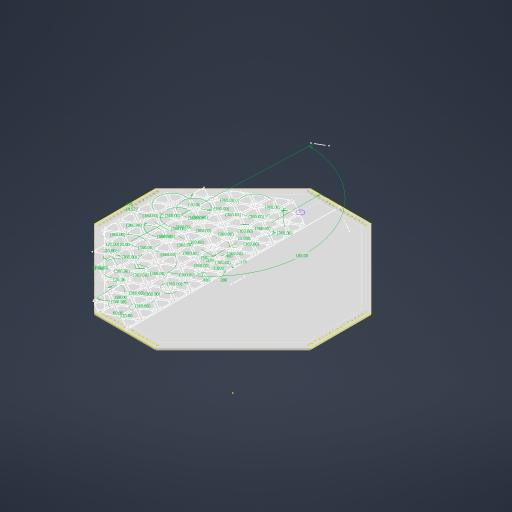
# Autodesk Inventor part: Belly Pan
Saved by Autodesk Inventor 2024.3 (Build 283343000, 343)
## iProperties
Created: 2024-11-27
Part Number: Belly Pan
Material: Generic
Document SubType Name: Modeling
Designer: kaito
Density: 1 g/cm^3
Appearance: Default
Author: kaito
Autodesk Inventor part; units mm, degrees
(part 1 of 3)
ref_plane "YZ Plane" through (0, 0, 0) normal (1, 0, 0) x (0, 1, 0)
ref_plane "XZ Plane" through (0, 0, 0) normal (0, 1, 0) x (-1, 0, 0)
ref_plane "XY Plane" through (0, 0, 0) normal (0, 0, 1) x (1, 0, 0)
sketch "Sketch1" plane through (0, 0, 0) normal (0, 1, 0) x (-1, 0, 0)
  line L0 (0, 0) -> (762, 0) construction
  line L1 (762, 0) -> (762, -762)
  line L2 (762, -762) -> (0, -762)
  line L3 (762, -273.05) -> (736.6, -273.05) construction
  line L4 (736.6, -273.05) -> (736.6, -488.95) construction
  line L5 (736.6, -488.95) -> (762, -488.95) construction
  line L6 (762, -488.95) -> (762, -273.05) construction
  line L7 (488.95, 0) -> (273.05, 0)
  line L8 (273.05, 0) -> (273.05, -25.4) construction
  line L9 (273.05, -25.4) -> (488.95, -25.4) construction
  line L10 (488.95, -25.4) -> (488.95, 0) construction
  line L11 (488.95, -762) -> (273.05, -762) construction
  line L12 (273.05, -762) -> (273.05, -736.6) construction
  line L13 (273.05, -736.6) -> (488.95, -736.6) construction
  line L14 (488.95, -736.6) -> (488.95, -762) construction
  line L15 (0, 0) -> (0, -762)
  line L16 (0, -273.05) -> (25.4, -273.05) construction
  line L17 (25.4, -273.05) -> (25.4, -488.95) construction
  line L18 (25.4, -488.95) -> (0, -488.95) construction
  line L19 (0, -488.95) -> (0, -273.05) construction
  line L20 (273.05, 0) -> (0, -273.05)
  line L21 (488.95, 0) -> (762, -273.05)
  line L22 (762, -488.95) -> (488.95, -762)
  line L23 (0, -488.95) -> (273.05, -762)
  circle A0 centre (482.6, -12.7) radius 2.4892
  circle A1 centre (469.9, -12.7) radius 2.4892
  circle A2 centre (457.2, -12.7) radius 2.4892
  circle A3 centre (444.5, -12.7) radius 2.4892
  circle A4 centre (431.8, -12.7) radius 2.4892
  circle A5 centre (419.1, -12.7) radius 2.4892
  circle A6 centre (406.4, -12.7) radius 2.4892
  circle A7 centre (393.7, -12.7) radius 2.4892
  circle A8 centre (381, -12.7) radius 2.4892
  circle A9 centre (368.3, -12.7) radius 2.4892
  circle A10 centre (355.6, -12.7) radius 2.4892
  circle A11 centre (342.9, -12.7) radius 2.4892
  circle A12 centre (330.2, -12.7) radius 2.4892
  circle A13 centre (317.5, -12.7) radius 2.4892
  circle A14 centre (304.8, -12.7) radius 2.4892
  circle A15 centre (292.1, -12.7) radius 2.4892
  circle A16 centre (279.4, -12.7) radius 2.4892
  circle A17 centre (749.3, -279.4) radius 2.4892
  circle A18 centre (749.3, -292.1) radius 2.4892
  circle A19 centre (749.3, -304.8) radius 2.4892
  circle A20 centre (749.3, -317.5) radius 2.4892
  circle A21 centre (749.3, -330.2) radius 2.4892
  circle A22 centre (749.3, -342.9) radius 2.4892
  circle A23 centre (749.3, -355.6) radius 2.4892
  circle A24 centre (749.3, -368.3) radius 2.4892
  circle A25 centre (749.3, -381) radius 2.4892
  circle A26 centre (749.3, -393.7) radius 2.4892
  circle A27 centre (749.3, -406.4) radius 2.4892
  circle A28 centre (749.3, -419.1) radius 2.4892
  circle A29 centre (749.3, -431.8) radius 2.4892
  circle A30 centre (749.3, -444.5) radius 2.4892
  circle A31 centre (749.3, -457.2) radius 2.4892
  circle A32 centre (749.3, -469.9) radius 2.4892
  circle A33 centre (749.3, -482.6) radius 2.4892
  circle A34 centre (482.6, -749.3) radius 2.4892
  circle A35 centre (469.9, -749.3) radius 2.4892
  circle A36 centre (457.2, -749.3) radius 2.4892
  circle A37 centre (444.5, -749.3) radius 2.4892
  circle A38 centre (431.8, -749.3) radius 2.4892
  circle A39 centre (419.1, -749.3) radius 2.4892
  circle A40 centre (406.4, -749.3) radius 2.4892
  circle A41 centre (393.7, -749.3) radius 2.4892
  circle A42 centre (381, -749.3) radius 2.4892
  circle A43 centre (368.3, -749.3) radius 2.4892
  circle A44 centre (355.6, -749.3) radius 2.4892
  circle A45 centre (342.9, -749.3) radius 2.4892
  circle A46 centre (330.2, -749.3) radius 2.4892
  circle A47 centre (317.5, -749.3) radius 2.4892
  circle A48 centre (304.8, -749.3) radius 2.4892
  circle A49 centre (292.1, -749.3) radius 2.4892
  circle A50 centre (279.4, -749.3) radius 2.4892
  circle A51 centre (12.7, -279.4) radius 2.4892
  circle A52 centre (12.7, -292.1) radius 2.4892
  circle A53 centre (12.7, -304.8) radius 2.4892
  circle A54 centre (12.7, -317.5) radius 2.4892
  circle A55 centre (12.7, -330.2) radius 2.4892
  circle A56 centre (12.7, -342.9) radius 2.4892
  circle A57 centre (12.7, -355.6) radius 2.4892
  circle A58 centre (12.7, -368.3) radius 2.4892
  circle A59 centre (12.7, -381) radius 2.4892
  circle A60 centre (12.7, -393.7) radius 2.4892
  circle A61 centre (12.7, -406.4) radius 2.4892
  circle A62 centre (12.7, -419.1) radius 2.4892
  circle A63 centre (12.7, -431.8) radius 2.4892
  circle A64 centre (12.7, -444.5) radius 2.4892
  circle A65 centre (12.7, -457.2) radius 2.4892
  circle A66 centre (12.7, -469.9) radius 2.4892
  circle A67 centre (12.7, -482.6) radius 2.4892
  point P0 (736.6, -381)
  point P1 (381, -25.4)
  point P2 (381, 0)
  point P3 (381, -736.6)
  point P4 (381, -762)
  point P5 (25.4, -381)
  point P6 (0, -381)
  point P7 (762, -381)
  point P8 (12.7, -273.05)
  point P9 (12.7, -488.95)
  point P10 (488.95, -12.7)
  point P11 (749.3, -273.05)
  point P12 (488.95, -749.3)
  point P13 (273.05, -762)
  point P14 (762, -488.95)
  point P15 (0, -381)
  dimension "d0" = 762
  dimension "d1" = 762
  dimension "d4" = 25.4
  dimension "d5" = 215.9
  dimension "d6" = 25.4
  dimension "d7" = 215.9
  dimension "d8" = 25.4
  dimension "d9" = 25.4
  dimension "d11" = 215.9
  dimension "d22" = 4.9784
  dimension "d23" = 6.35
  dimension "d26" = 12.7
  dimension "d31" = 4.9784
  dimension "d32" = 6.35
  dimension "d35" = 12.7
  dimension "d40" = 4.9784
  dimension "d41" = 6.35
  dimension "d44" = 12.7
  dimension "d51" = 215.9
  dimension "d60" = 4.9784
  dimension "d63" = 12.7
  constraints: 68 centre point, 48 end point, 14 midpoint, 9 parallel, 7 horizontal, 5 horizontal alignment, 5 perpendicular, 4 point on line, 4 vertical alignment, 3 vertical, 128 other
  measures "d0" distance of L1.end L2.end
  measures "d1" distance of L0.end L1.end
  measures "d4" distance of L5.end L4.end
  measures "d5" distance of L9.end L8.end
  measures "d6" distance of L8.end L7.end
  measures "d7" distance of L12.end L13.end
  measures "d8" distance of L11.end L12.end
  measures "d9" distance of L17.end L18.end
  measures "d11" distance of L3.end L4.end
  measures "d22" diameter of A0
  measures "d23" distance from line of L10 A0.centre
  measures "d26" distance of A0.centre A1.centre
  measures "d31" diameter of A17
  measures "d32" distance of point (749.3, -273.05) A17.centre
  measures "d35" distance of A17.centre A18.centre
  measures "d40" diameter of A34
  measures "d41" distance of A34.centre point (488.95, -749.3)
  measures "d44" distance of A34.centre A35.centre
  measures "d51" distance of L16.end L17.end
  measures "d60" diameter of A51
  measures "d63" distance of A51.centre A52.centre
extrude "Extrusion1" add sketch "Sketch1" along normal blind 6.35 contours L1 L22 L2 L23 L15 L20 L7 L21
sketch "Sketch4" plane through (0, 6.35, 0) normal (0, 1, 0) x (1, 0, 0)
  line L0 (-762, 488.95) -> (-762, 273.05) projected
  line L1 (0, 273.05) -> (0, 488.95) projected
  line L2 (-488.95, 0) -> (-273.05, 0) projected
  line L3 (-381, 0) -> (-381, 762)
  line L4 (-273.05, 762) -> (-488.95, 762) projected
  circle A0 centre (-432.435, 381) radius 11.43 construction
  line L5 (-393.065, 361.9359) -> (-418.465, 376.6006)
  line L6 (-418.465, 385.3994) -> (-393.065, 400.0641)
  line L7 (-385.445, 395.6647) -> (-385.445, 366.3353)
  arc A1 (-393.065, 361.9359) -> (-385.445, 366.3353) centre (-390.525, 366.3353) ccw
  arc A2 (-418.465, 385.3994) -> (-418.465, 376.6006) centre (-415.925, 381) ccw
  arc A3 (-385.445, 395.6647) -> (-393.065, 400.0641) centre (-390.525, 395.6647) ccw
  circle A4 centre (-432.435, 381) radius 11.43 construction
  arc A5 (-429.26, 395.2981) -> (-421.64, 390.8987) centre (-424.18, 395.2981) ccw
  line L8 (-396.24, 405.5634) -> (-421.64, 390.8987)
  arc A6 (-396.24, 405.5634) -> (-396.24, 414.3622) centre (-398.78, 409.9628) ccw
  arc A7 (-421.64, 429.0269) -> (-429.26, 424.6275) centre (-424.18, 424.6275) ccw
  line L9 (-429.26, 395.2981) -> (-429.26, 424.6275)
  line L10 (-421.64, 429.0269) -> (-396.24, 414.3622)
  circle A8 centre (-432.435, 381) radius 11.43 construction
  arc A9 (-443.23, 390.8987) -> (-435.61, 395.2981) centre (-440.69, 395.2981) ccw
  line L11 (-435.61, 424.6275) -> (-435.61, 395.2981)
  arc A10 (-435.61, 424.6275) -> (-443.23, 429.0269) centre (-440.69, 424.6275) ccw
  arc A11 (-468.63, 414.3622) -> (-468.63, 405.5634) centre (-466.09, 409.9628) ccw
  line L12 (-443.23, 390.8987) -> (-468.63, 405.5634)
  line L13 (-468.63, 414.3622) -> (-443.23, 429.0269)
  circle A12 centre (-432.435, 381) radius 11.43 construction
  arc A13 (-446.405, 376.6006) -> (-446.405, 385.3994) centre (-448.945, 381) ccw
  line L14 (-471.805, 400.0641) -> (-446.405, 385.3994)
  arc A14 (-471.805, 400.0641) -> (-479.425, 395.6647) centre (-474.345, 395.6647) ccw
  arc A15 (-479.425, 366.3353) -> (-471.805, 361.9359) centre (-474.345, 366.3353) ccw
  line L15 (-446.405, 376.6006) -> (-471.805, 361.9359)
  line L16 (-479.425, 366.3353) -> (-479.425, 395.6647)
  circle A16 centre (-432.435, 381) radius 11.43 construction
  arc A17 (-435.61, 366.7019) -> (-443.23, 371.1013) centre (-440.69, 366.7019) ccw
  line L17 (-468.63, 356.4366) -> (-443.23, 371.1013)
  arc A18 (-468.63, 356.4366) -> (-468.63, 347.6378) centre (-466.09, 352.0372) ccw
  arc A19 (-443.23, 332.9731) -> (-435.61, 337.3725) centre (-440.69, 337.3725) ccw
  line L18 (-435.61, 366.7019) -> (-435.61, 337.3725)
  line L19 (-443.23, 332.9731) -> (-468.63, 347.6378)
  circle A20 centre (-432.435, 381) radius 11.43 construction
  arc A21 (-421.64, 371.1013) -> (-429.26, 366.7019) centre (-424.18, 366.7019) ccw
  line L20 (-429.26, 337.3725) -> (-429.26, 366.7019)
  arc A22 (-429.26, 337.3725) -> (-421.64, 332.9731) centre (-424.18, 337.3725) ccw
  arc A23 (-396.24, 347.6378) -> (-396.24, 356.4366) centre (-398.78, 352.0372) ccw
  line L21 (-421.64, 371.1013) -> (-396.24, 356.4366)
  line L22 (-396.24, 347.6378) -> (-421.64, 332.9731)
  circle A24 centre (-432.435, 381) radius 5.08
  circle A25 centre (-749.9958, 381) radius 6.3038 construction
  line L23 (-432.435, 381) -> (-432.435, 762) construction
  line L24 (-749.9958, 381) -> (-381, 381) construction
  circle A26 centre (-432.435, 323.0744) radius 11.43 construction
  line L25 (-446.405, 318.675) -> (-471.805, 304.0103)
  arc A27 (-446.405, 318.675) -> (-446.405, 327.4739) centre (-448.945, 323.0744) ccw
  line L26 (-471.805, 342.1386) -> (-446.405, 327.4739)
  arc A28 (-471.805, 342.1386) -> (-479.425, 337.7391) centre (-474.345, 337.7391) ccw
  line L27 (-479.425, 308.4098) -> (-479.425, 337.7391)
  arc A29 (-479.425, 308.4098) -> (-471.805, 304.0103) centre (-474.345, 308.4098) ccw
  line L28 (-435.61, 308.7764) -> (-435.61, 279.447)
  arc A30 (-435.61, 308.7764) -> (-443.23, 313.1758) centre (-440.69, 308.7764) ccw
  line L29 (-468.63, 298.5111) -> (-443.23, 313.1758)
  arc A31 (-468.63, 298.5111) -> (-468.63, 289.7123) centre (-466.09, 294.1117) ccw
  line L30 (-443.23, 275.0476) -> (-468.63, 289.7123)
  arc A32 (-443.23, 275.0476) -> (-435.61, 279.447) centre (-440.69, 279.447) ccw
  line L31 (-421.64, 313.1758) -> (-396.24, 298.5111)
  arc A33 (-421.64, 313.1758) -> (-429.26, 308.7764) centre (-424.18, 308.7764) ccw
  line L32 (-429.26, 279.447) -> (-429.26, 308.7764)
  arc A34 (-429.26, 279.447) -> (-421.64, 275.0476) centre (-424.18, 279.447) ccw
  line L33 (-396.24, 289.7123) -> (-421.64, 275.0476)
  arc A35 (-396.24, 289.7123) -> (-396.24, 298.5111) centre (-398.78, 294.1117) ccw
  line L34 (-418.465, 327.4739) -> (-393.065, 342.1386)
  arc A36 (-418.465, 327.4739) -> (-418.465, 318.675) centre (-415.925, 323.0744) ccw
  line L35 (-393.065, 304.0103) -> (-418.465, 318.675)
  arc A37 (-393.065, 304.0103) -> (-385.445, 308.4098) centre (-390.525, 308.4098) ccw
  line L36 (-385.445, 337.7391) -> (-385.445, 308.4098)
  arc A38 (-385.445, 337.7391) -> (-393.065, 342.1386) centre (-390.525, 337.7391) ccw
  line L37 (-429.26, 337.3725) -> (-429.26, 366.7019)
  arc A39 (-429.26, 337.3725) -> (-421.64, 332.9731) centre (-424.18, 337.3725) ccw
  line L38 (-396.24, 347.6378) -> (-421.64, 332.9731)
  arc A40 (-396.24, 347.6378) -> (-396.24, 356.4366) centre (-398.78, 352.0372) ccw
  line L39 (-421.64, 371.1013) -> (-396.24, 356.4366)
  arc A41 (-421.64, 371.1013) -> (-429.26, 366.7019) centre (-424.18, 366.7019) ccw
  circle A42 centre (-432.435, 323.0744) radius 5.08
  line L40 (-273.05, 0) -> (0, 273.05) construction
  line L41 (0, 273.05) -> (0, 488.95) construction
  line L42 (0, 488.95) -> (-273.05, 762) construction
  line L43 (-273.05, 762) -> (-488.95, 762) construction
  line L44 (-488.95, 762) -> (-762, 488.95) construction
  line L45 (-762, 488.95) -> (-762, 273.05) construction
  line L46 (-762, 273.05) -> (-488.95, 0) construction
  line L47 (-488.95, 0) -> (-273.05, 0) construction
  circle A43 centre (-12.7, 482.6) radius 2.4892 construction
  circle A44 centre (-12.7, 457.2) radius 2.4892 construction
  circle A45 centre (-12.7, 431.8) radius 2.4892 construction
  circle A46 centre (-12.7, 406.4) radius 2.4892 construction
  circle A47 centre (-12.7, 381) radius 2.4892 construction
  circle A48 centre (-12.7, 355.6) radius 2.4892 construction
  circle A49 centre (-12.7, 330.2) radius 2.4892 construction
  circle A50 centre (-12.7, 304.8) radius 2.4892 construction
  circle A51 centre (-12.7, 279.4) radius 2.4892 construction
  circle A52 centre (-292.1, 749.3) radius 2.4892 construction
  circle A53 centre (-317.5, 749.3) radius 2.4892 construction
  circle A54 centre (-342.9, 749.3) radius 2.4892 construction
  circle A55 centre (-368.3, 749.3) radius 2.4892 construction
  circle A56 centre (-393.7, 749.3) radius 2.4892 construction
  circle A57 centre (-419.1, 749.3) radius 2.4892 construction
  circle A58 centre (-444.5, 749.3) radius 2.4892 construction
  circle A59 centre (-469.9, 749.3) radius 2.4892 construction
  circle A60 centre (-749.3, 482.6) radius 2.4892 construction
  circle A61 centre (-749.3, 457.2) radius 2.4892 construction
  circle A62 centre (-749.3, 431.8) radius 2.4892 construction
  circle A63 centre (-749.3, 406.4) radius 2.4892 construction
  circle A64 centre (-749.3, 381) radius 2.4892 construction
  circle A65 centre (-749.3, 355.6) radius 2.4892 construction
  circle A66 centre (-749.3, 330.2) radius 2.4892 construction
  circle A67 centre (-749.3, 304.8) radius 2.4892 construction
  circle A68 centre (-749.3, 279.4) radius 2.4892 construction
  circle A69 centre (-292.1, 12.7) radius 2.4892 construction
  circle A70 centre (-317.5, 12.7) radius 2.4892 construction
  circle A71 centre (-342.9, 12.7) radius 2.4892 construction
  circle A72 centre (-368.3, 12.7) radius 2.4892 construction
  circle A73 centre (-393.7, 12.7) radius 2.4892 construction
  circle A74 centre (-482.6, 12.7) radius 2.4892 construction
  circle A75 centre (-469.9, 12.7) radius 2.4892 construction
  circle A76 centre (-457.2, 12.7) radius 2.4892 construction
  circle A77 centre (-444.5, 12.7) radius 2.4892 construction
  circle A78 centre (-431.8, 12.7) radius 2.4892 construction
  circle A79 centre (-419.1, 12.7) radius 2.4892 construction
  circle A80 centre (-406.4, 12.7) radius 2.4892 construction
  circle A81 centre (-381, 12.7) radius 2.4892 construction
  circle A82 centre (-355.6, 12.7) radius 2.4892 construction
  circle A83 centre (-330.2, 12.7) radius 2.4892 construction
  circle A84 centre (-304.8, 12.7) radius 2.4892 construction
  circle A85 centre (-279.4, 12.7) radius 2.4892 construction
  circle A86 centre (-749.3, 292.1) radius 2.4892 construction
  circle A87 centre (-749.3, 317.5) radius 2.4892 construction
  circle A88 centre (-749.3, 342.9) radius 2.4892 construction
  circle A89 centre (-749.3, 368.3) radius 2.4892 construction
  circle A90 centre (-749.3, 393.7) radius 2.4892 construction
  circle A91 centre (-749.3, 419.1) radius 2.4892 construction
  circle A92 centre (-749.3, 444.5) radius 2.4892 construction
  circle A93 centre (-749.3, 469.9) radius 2.4892 construction
  circle A94 centre (-482.6, 749.3) radius 2.4892 construction
  circle A95 centre (-457.2, 749.3) radius 2.4892 construction
  circle A96 centre (-431.8, 749.3) radius 2.4892 construction
  circle A97 centre (-406.4, 749.3) radius 2.4892 construction
  circle A98 centre (-381, 749.3) radius 2.4892 construction
  circle A99 centre (-355.6, 749.3) radius 2.4892 construction
  circle A100 centre (-330.2, 749.3) radius 2.4892 construction
  circle A101 centre (-304.8, 749.3) radius 2.4892 construction
  circle A102 centre (-279.4, 749.3) radius 2.4892 construction
  circle A103 centre (-12.7, 292.1) radius 2.4892 construction
  circle A104 centre (-12.7, 317.5) radius 2.4892 construction
  circle A105 centre (-12.7, 342.9) radius 2.4892 construction
  circle A106 centre (-12.7, 368.3) radius 2.4892 construction
  circle A107 centre (-12.7, 393.7) radius 2.4892 construction
  circle A108 centre (-12.7, 419.1) radius 2.4892 construction
  circle A109 centre (-12.7, 444.5) radius 2.4892 construction
  circle A110 centre (-12.7, 469.9) radius 2.4892 construction
  line L48 (-478.429, 25.4) -> (-736.6, 283.571)
  line L49 (-736.6, 283.571) -> (-736.6, 478.429) construction
  line L50 (-736.6, 478.429) -> (-478.429, 736.6) construction
  line L51 (-478.429, 736.6) -> (-283.571, 736.6) construction
  line L52 (-283.571, 736.6) -> (-25.4, 478.429) construction
  line L53 (-25.4, 478.429) -> (-25.4, 283.571) construction
  line L54 (-25.4, 283.571) -> (-283.571, 25.4) construction
  line L55 (-283.571, 25.4) -> (-478.429, 25.4) construction
  circle A111 centre (-432.435, 265.1489) radius 11.43 construction
  arc A112 (-446.405, 260.7495) -> (-446.405, 269.5483) centre (-448.945, 265.1489) ccw
  line L56 (-471.805, 284.213) -> (-446.405, 269.5483)
  arc A113 (-471.805, 284.213) -> (-479.425, 279.8136) centre (-474.345, 279.8136) ccw
  line L57 (-479.425, 250.4842) -> (-479.425, 279.8136)
  line L58 (-446.405, 260.7495) -> (-471.805, 246.0848)
  arc A114 (-479.425, 250.4842) -> (-471.805, 246.0848) centre (-474.345, 250.4842) ccw
  arc A115 (-435.61, 250.8508) -> (-443.23, 255.2502) centre (-440.69, 250.8508) ccw
  line L59 (-468.63, 240.5855) -> (-443.23, 255.2502)
  arc A116 (-468.63, 240.5855) -> (-468.63, 231.7867) centre (-466.09, 236.1861) ccw
  line L60 (-443.23, 217.122) -> (-468.63, 231.7867)
  line L61 (-435.61, 250.8508) -> (-435.61, 221.5214)
  arc A117 (-443.23, 217.122) -> (-435.61, 221.5214) centre (-440.69, 221.5214) ccw
  arc A118 (-421.64, 255.2502) -> (-429.26, 250.8508) centre (-424.18, 250.8508) ccw
  line L62 (-429.26, 221.5214) -> (-429.26, 250.8508)
  arc A119 (-429.26, 221.5214) -> (-421.64, 217.122) centre (-424.18, 221.5214) ccw
  line L63 (-396.24, 231.7867) -> (-421.64, 217.122)
  line L64 (-421.64, 255.2502) -> (-396.24, 240.5855)
  arc A120 (-396.24, 231.7867) -> (-396.24, 240.5855) centre (-398.78, 236.1861) ccw
  arc A121 (-418.465, 269.5483) -> (-418.465, 260.7495) centre (-415.925, 265.1489) ccw
  line L65 (-393.065, 246.0848) -> (-418.465, 260.7495)
  arc A122 (-393.065, 246.0848) -> (-385.445, 250.4842) centre (-390.525, 250.4842) ccw
  line L66 (-385.445, 279.8136) -> (-385.445, 250.4842)
  line L67 (-418.465, 269.5483) -> (-393.065, 284.213)
  arc A123 (-385.445, 279.8136) -> (-393.065, 284.213) centre (-390.525, 279.8136) ccw
  arc A124 (-429.26, 279.447) -> (-421.64, 275.0476) centre (-424.18, 279.447) ccw
  line L68 (-396.24, 289.7123) -> (-421.64, 275.0476)
  arc A125 (-396.24, 289.7123) -> (-396.24, 298.5111) centre (-398.78, 294.1117) ccw
  line L69 (-421.64, 313.1758) -> (-396.24, 298.5111)
  line L70 (-429.26, 279.447) -> (-429.26, 308.7764)
  arc A126 (-421.64, 313.1758) -> (-429.26, 308.7764) centre (-424.18, 308.7764) ccw
  circle A127 centre (-432.435, 207.2233) radius 11.43 construction
  line L71 (-471.805, 226.2874) -> (-446.405, 211.6228)
  arc A128 (-446.405, 202.8239) -> (-446.405, 211.6228) centre (-448.945, 207.2233) ccw
  line L72 (-446.405, 202.8239) -> (-471.805, 188.1592)
  arc A129 (-479.425, 192.5586) -> (-471.805, 188.1592) centre (-474.345, 192.5586) ccw
  line L73 (-479.425, 192.5586) -> (-479.425, 221.888)
  arc A130 (-471.805, 226.2874) -> (-479.425, 221.888) centre (-474.345, 221.888) ccw
  line L74 (-468.63, 182.66) -> (-443.23, 197.3247)
  arc A131 (-435.61, 192.9253) -> (-443.23, 197.3247) centre (-440.69, 192.9253) ccw
  line L75 (-435.61, 192.9253) -> (-435.61, 163.5959)
  arc A132 (-443.23, 159.1965) -> (-435.61, 163.5959) centre (-440.69, 163.5959) ccw
  line L76 (-443.23, 159.1965) -> (-468.63, 173.8612)
  arc A133 (-468.63, 182.66) -> (-468.63, 173.8612) centre (-466.09, 178.2606) ccw
  line L77 (-429.26, 163.5959) -> (-429.26, 192.9253)
  arc A134 (-421.64, 197.3247) -> (-429.26, 192.9253) centre (-424.18, 192.9253) ccw
  line L78 (-421.64, 197.3247) -> (-396.24, 182.66)
  arc A135 (-396.24, 173.8612) -> (-396.24, 182.66) centre (-398.78, 178.2606) ccw
  line L79 (-396.24, 173.8612) -> (-421.64, 159.1965)
  arc A136 (-429.26, 163.5959) -> (-421.64, 159.1965) centre (-424.18, 163.5959) ccw
  line L80 (-393.065, 188.1592) -> (-418.465, 202.8239)
  arc A137 (-418.465, 211.6228) -> (-418.465, 202.8239) centre (-415.925, 207.2233) ccw
  line L81 (-418.465, 211.6228) -> (-393.065, 226.2874)
  arc A138 (-385.445, 221.888) -> (-393.065, 226.2874) centre (-390.525, 221.888) ccw
  line L82 (-385.445, 221.888) -> (-385.445, 192.5586)
  arc A139 (-393.065, 188.1592) -> (-385.445, 192.5586) centre (-390.525, 192.5586) ccw
  line L83 (-396.24, 231.7867) -> (-421.64, 217.122)
  arc A140 (-429.26, 221.5214) -> (-421.64, 217.122) centre (-424.18, 221.5214) ccw
  line L84 (-429.26, 221.5214) -> (-429.26, 250.8508)
  arc A141 (-421.64, 255.2502) -> (-429.26, 250.8508) centre (-424.18, 250.8508) ccw
  line L85 (-421.64, 255.2502) -> (-396.24, 240.5855)
  arc A142 (-396.24, 231.7867) -> (-396.24, 240.5855) centre (-398.78, 236.1861) ccw
  circle A143 centre (-432.435, 149.2978) radius 11.43 construction
  line L86 (-446.405, 144.8984) -> (-471.805, 130.2337)
  arc A144 (-446.405, 144.8984) -> (-446.405, 153.6972) centre (-448.945, 149.2978) ccw
  line L87 (-471.805, 168.3619) -> (-446.405, 153.6972)
  arc A145 (-471.805, 168.3619) -> (-479.425, 163.9625) centre (-474.345, 163.9625) ccw
  line L88 (-479.425, 134.6331) -> (-479.425, 163.9625)
  arc A146 (-479.425, 134.6331) -> (-471.805, 130.2337) centre (-474.345, 134.6331) ccw
  line L89 (-435.61, 134.9997) -> (-435.61, 105.6703)
  arc A147 (-435.61, 134.9997) -> (-443.23, 139.3991) centre (-440.69, 134.9997) ccw
  line L90 (-468.63, 124.7344) -> (-443.23, 139.3991)
  arc A148 (-468.63, 124.7344) -> (-468.63, 115.9356) centre (-466.09, 120.335) ccw
  line L91 (-443.23, 101.2709) -> (-468.63, 115.9356)
  arc A149 (-443.23, 101.2709) -> (-435.61, 105.6703) centre (-440.69, 105.6703) ccw
  line L92 (-421.64, 139.3991) -> (-396.24, 124.7344)
  arc A150 (-421.64, 139.3991) -> (-429.26, 134.9997) centre (-424.18, 134.9997) ccw
  line L93 (-429.26, 105.6703) -> (-429.26, 134.9997)
  arc A151 (-429.26, 105.6703) -> (-421.64, 101.2709) centre (-424.18, 105.6703) ccw
  line L94 (-396.24, 115.9356) -> (-421.64, 101.2709)
  arc A152 (-396.24, 115.9356) -> (-396.24, 124.7344) centre (-398.78, 120.335) ccw
  line L95 (-418.465, 153.6972) -> (-393.065, 168.3619)
  arc A153 (-418.465, 153.6972) -> (-418.465, 144.8984) centre (-415.925, 149.2978) ccw
  line L96 (-393.065, 130.2337) -> (-418.465, 144.8984)
  arc A154 (-393.065, 130.2337) -> (-385.445, 134.6331) centre (-390.525, 134.6331) ccw
  line L97 (-385.445, 163.9625) -> (-385.445, 134.6331)
  arc A155 (-385.445, 163.9625) -> (-393.065, 168.3619) centre (-390.525, 163.9625) ccw
  line L98 (-429.26, 163.5959) -> (-429.26, 192.9253)
  arc A156 (-429.26, 163.5959) -> (-421.64, 159.1965) centre (-424.18, 163.5959) ccw
  line L99 (-396.24, 173.8612) -> (-421.64, 159.1965)
  arc A157 (-396.24, 173.8612) -> (-396.24, 182.66) centre (-398.78, 178.2606) ccw
  line L100 (-421.64, 197.3247) -> (-396.24, 182.66)
  arc A158 (-421.64, 197.3247) -> (-429.26, 192.9253) centre (-424.18, 192.9253) ccw
  circle A159 centre (-432.435, 91.3722) radius 11.43 construction
  arc A160 (-443.23, 101.2709) -> (-435.61, 105.6703) centre (-440.69, 105.6703) ccw
  line L101 (-435.61, 134.9997) -> (-435.61, 105.6703)
  arc A161 (-435.61, 134.9997) -> (-443.23, 139.3991) centre (-440.69, 134.9997) ccw
  line L102 (-468.63, 124.7344) -> (-443.23, 139.3991)
  line L103 (-443.23, 101.2709) -> (-468.63, 115.9356)
  arc A162 (-468.63, 124.7344) -> (-468.63, 115.9356) centre (-466.09, 120.335) ccw
  arc A163 (-446.405, 86.9728) -> (-446.405, 95.7716) centre (-448.945, 91.3722) ccw
  line L104 (-471.805, 110.4363) -> (-446.405, 95.7716)
  arc A164 (-471.805, 110.4363) -> (-479.425, 106.0369) centre (-474.345, 106.0369) ccw
  line L105 (-479.425, 76.7075) -> (-479.425, 106.0369)
  line L106 (-446.405, 86.9728) -> (-471.805, 72.3081)
  arc A165 (-479.425, 76.7075) -> (-471.805, 72.3081) centre (-474.345, 76.7075) ccw
  arc A166 (-435.61, 77.0742) -> (-443.23, 81.4736) centre (-440.69, 77.0742) ccw
  line L107 (-468.63, 66.8089) -> (-443.23, 81.4736)
  arc A167 (-468.63, 66.8089) -> (-468.63, 58.0101) centre (-466.09, 62.4095) ccw
  line L108 (-443.23, 43.3454) -> (-468.63, 58.0101)
  line L109 (-435.61, 77.0742) -> (-435.61, 47.7448)
  arc A168 (-443.23, 43.3454) -> (-435.61, 47.7448) centre (-440.69, 47.7448) ccw
  arc A169 (-421.64, 81.4736) -> (-429.26, 77.0742) centre (-424.18, 77.0742) ccw
  line L110 (-429.26, 47.7448) -> (-429.26, 77.0742)
  arc A170 (-429.26, 47.7448) -> (-421.64, 43.3454) centre (-424.18, 47.7448) ccw
  line L111 (-396.24, 58.0101) -> (-421.64, 43.3454)
  line L112 (-421.64, 81.4736) -> (-396.24, 66.8089)
  arc A171 (-396.24, 58.0101) -> (-396.24, 66.8089) centre (-398.78, 62.4095) ccw
  arc A172 (-418.465, 95.7716) -> (-418.465, 86.9728) centre (-415.925, 91.3722) ccw
  line L113 (-393.065, 72.3081) -> (-418.465, 86.9728)
  arc A173 (-393.065, 72.3081) -> (-385.445, 76.7075) centre (-390.525, 76.7075) ccw
  line L114 (-385.445, 106.0369) -> (-385.445, 76.7075)
  line L115 (-418.465, 95.7716) -> (-393.065, 110.4363)
  arc A174 (-385.445, 106.0369) -> (-393.065, 110.4363) centre (-390.525, 106.0369) ccw
  circle A175 centre (-432.435, 33.4467) radius 11.43 construction
  arc A176 (-418.465, 37.8461) -> (-418.465, 29.0473) centre (-415.925, 33.4467) ccw
  line L116 (-418.465, 37.8461) -> (-393.065, 52.5108)
  arc A177 (-385.445, 48.1114) -> (-393.065, 52.5108) centre (-390.525, 48.1114) ccw
  line L117 (-385.445, 48.1114) -> (-385.445, 18.782)
  arc A178 (-393.065, 14.3826) -> (-385.445, 18.782) centre (-390.525, 18.782) ccw
  line L118 (-393.065, 14.3826) -> (-418.465, 29.0473)
  arc A179 (-446.405, 29.0473) -> (-446.405, 37.8461) centre (-448.945, 33.4467) ccw
  line L119 (-446.405, 29.0473) -> (-471.805, 14.3826)
  arc A180 (-479.425, 18.782) -> (-471.805, 14.3826) centre (-474.345, 18.782) ccw
  line L120 (-479.425, 18.782) -> (-479.425, 48.1114)
  arc A181 (-471.805, 52.5108) -> (-479.425, 48.1114) centre (-474.345, 48.1114) ccw
  line L121 (-471.805, 52.5108) -> (-446.405, 37.8461)
  circle A182 centre (-482.6, 62.4095) radius 11.43 construction
  line L122 (-493.395, 72.3081) -> (-518.795, 86.9728)
  arc A183 (-493.395, 72.3081) -> (-485.775, 76.7075) centre (-490.855, 76.7075) ccw
  line L123 (-485.775, 106.0369) -> (-485.775, 76.7075)
  arc A184 (-485.775, 106.0369) -> (-493.395, 110.4363) centre (-490.855, 106.0369) ccw
  arc A185 (-518.795, 95.7716) -> (-518.795, 86.9728) centre (-516.255, 91.3722) ccw
  line L124 (-518.795, 95.7716) -> (-493.395, 110.4363)
  line L125 (-496.57, 58.0101) -> (-521.97, 43.3454)
  arc A186 (-496.57, 58.0101) -> (-496.57, 66.8089) centre (-499.11, 62.4095) ccw
  line L126 (-521.97, 81.4736) -> (-496.57, 66.8089)
  arc A187 (-521.97, 81.4736) -> (-529.59, 77.0742) centre (-524.51, 77.0742) ccw
  arc A188 (-529.59, 47.7448) -> (-521.97, 43.3454) centre (-524.51, 47.7448) ccw
  line L127 (-529.59, 47.7448) -> (-529.59, 77.0742)
  line L128 (-485.775, 48.1114) -> (-485.775, 18.782)
  arc A189 (-485.775, 48.1114) -> (-493.395, 52.5108) centre (-490.855, 48.1114) ccw
  line L129 (-518.795, 37.8461) -> (-493.395, 52.5108)
  arc A190 (-518.795, 37.8461) -> (-518.795, 29.0473) centre (-516.255, 33.4467) ccw
  arc A191 (-493.395, 14.3826) -> (-485.775, 18.782) centre (-490.855, 18.782) ccw
  line L130 (-493.395, 14.3826) -> (-518.795, 29.0473)
  line L131 (-471.805, 52.5108) -> (-446.405, 37.8461)
  arc A192 (-471.805, 52.5108) -> (-479.425, 48.1114) centre (-474.345, 48.1114) ccw
  line L132 (-479.425, 18.782) -> (-479.425, 48.1114)
  arc A193 (-479.425, 18.782) -> (-471.805, 14.3826) centre (-474.345, 18.782) ccw
  arc A194 (-446.405, 29.0473) -> (-446.405, 37.8461) centre (-448.945, 33.4467) ccw
  line L133 (-446.405, 29.0473) -> (-471.805, 14.3826)
  line L134 (-468.63, 66.8089) -> (-443.23, 81.4736)
  arc A195 (-468.63, 66.8089) -> (-468.63, 58.0101) centre (-466.09, 62.4095) ccw
  line L135 (-443.23, 43.3454) -> (-468.63, 58.0101)
  arc A196 (-443.23, 43.3454) -> (-435.61, 47.7448) centre (-440.69, 47.7448) ccw
  arc A197 (-435.61, 77.0742) -> (-443.23, 81.4736) centre (-440.69, 77.0742) ccw
  line L136 (-435.61, 77.0742) -> (-435.61, 47.7448)
  circle A198 centre (-482.6, 120.335) radius 11.43 construction
  arc A199 (-493.395, 130.2337) -> (-485.775, 134.6331) centre (-490.855, 134.6331) ccw
  line L137 (-493.395, 130.2337) -> (-518.795, 144.8984)
  arc A200 (-518.795, 153.6972) -> (-518.795, 144.8984) centre (-516.255, 149.2978) ccw
  line L138 (-518.795, 153.6972) -> (-493.395, 168.3619)
  circle A201 centre (-482.6, 178.2606) radius 11.43 construction
  line L139 (-485.775, 163.9625) -> (-485.775, 134.6331)
  arc A202 (-485.775, 163.9625) -> (-493.395, 168.3619) centre (-490.855, 163.9625) ccw
  arc A203 (-496.57, 115.9356) -> (-496.57, 124.7344) centre (-499.11, 120.335) ccw
  line L140 (-496.57, 115.9356) -> (-521.97, 101.2709)
  arc A204 (-529.59, 105.6703) -> (-521.97, 101.2709) centre (-524.51, 105.6703) ccw
  line L141 (-529.59, 105.6703) -> (-529.59, 134.9997)
  circle A205 centre (-532.765, 149.2978) radius 11.43 construction
  line L142 (-521.97, 139.3991) -> (-496.57, 124.7344)
  arc A206 (-521.97, 139.3991) -> (-529.59, 134.9997) centre (-524.51, 134.9997) ccw
  arc A207 (-485.775, 106.0369) -> (-493.395, 110.4363) centre (-490.855, 106.0369) ccw
  line L143 (-485.775, 106.0369) -> (-485.775, 76.7075)
  arc A208 (-493.395, 72.3081) -> (-485.775, 76.7075) centre (-490.855, 76.7075) ccw
  line L144 (-493.395, 72.3081) -> (-518.795, 86.9728)
  circle A209 centre (-532.765, 91.3722) radius 11.43 construction
  line L145 (-518.795, 95.7716) -> (-493.395, 110.4363)
  arc A210 (-518.795, 95.7716) -> (-518.795, 86.9728) centre (-516.255, 91.3722) ccw
  arc A211 (-471.805, 110.4363) -> (-479.425, 106.0369) centre (-474.345, 106.0369) ccw
  line L146 (-471.805, 110.4363) -> (-446.405, 95.7716)
  arc A212 (-446.405, 86.9728) -> (-446.405, 95.7716) centre (-448.945, 91.3722) ccw
  line L147 (-446.405, 86.9728) -> (-471.805, 72.3081)
  circle A213 centre (-482.6, 62.4095) radius 11.43 construction
  line L148 (-479.425, 76.7075) -> (-479.425, 106.0369)
  arc A214 (-479.425, 76.7075) -> (-471.805, 72.3081) centre (-474.345, 76.7075) ccw
  arc A215 (-468.63, 124.7344) -> (-468.63, 115.9356) centre (-466.09, 120.335) ccw
  line L149 (-468.63, 124.7344) -> (-443.23, 139.3991)
  arc A216 (-435.61, 134.9997) -> (-443.23, 139.3991) centre (-440.69, 134.9997) ccw
  line L150 (-435.61, 134.9997) -> (-435.61, 105.6703)
  circle A217 centre (-432.435, 91.3722) radius 11.43 construction
  line L151 (-443.23, 101.2709) -> (-468.63, 115.9356)
  arc A218 (-443.23, 101.2709) -> (-435.61, 105.6703) centre (-440.69, 105.6703) ccw
  line L152 (-493.395, 72.3081) -> (-518.795, 86.9728)
  arc A219 (-493.395, 72.3081) -> (-485.775, 76.7075) centre (-490.855, 76.7075) ccw
  line L153 (-485.775, 106.0369) -> (-485.775, 76.7075)
  arc A220 (-485.775, 106.0369) -> (-493.395, 110.4363) centre (-490.855, 106.0369) ccw
  line L154 (-518.795, 95.7716) -> (-493.395, 110.4363)
  arc A221 (-518.795, 95.7716) -> (-518.795, 86.9728) centre (-516.255, 91.3722) ccw
  line L155 (-496.57, 115.9356) -> (-521.97, 101.2709)
  arc A222 (-496.57, 115.9356) -> (-496.57, 124.7344) centre (-499.11, 120.335) ccw
  line L156 (-521.97, 139.3991) -> (-496.57, 124.7344)
  arc A223 (-521.97, 139.3991) -> (-529.59, 134.9997) centre (-524.51, 134.9997) ccw
  line L157 (-529.59, 105.6703) -> (-529.59, 134.9997)
  arc A224 (-529.59, 105.6703) -> (-521.97, 101.2709) centre (-524.51, 105.6703) ccw
  line L158 (-535.94, 134.9997) -> (-535.94, 105.6703)
  arc A225 (-535.94, 134.9997) -> (-543.56, 139.3991) centre (-541.02, 134.9997) ccw
  line L159 (-568.96, 124.7344) -> (-543.56, 139.3991)
  arc A226 (-568.96, 124.7344) -> (-568.96, 115.9356) centre (-566.42, 120.335) ccw
  line L160 (-543.56, 101.2709) -> (-568.96, 115.9356)
  arc A227 (-543.56, 101.2709) -> (-535.94, 105.6703) centre (-541.02, 105.6703) ccw
  circle A228 centre (-582.93, 120.335) radius 11.43 construction
  line L161 (-546.735, 144.8984) -> (-572.135, 130.2337)
  arc A229 (-546.735, 144.8984) -> (-546.735, 153.6972) centre (-549.275, 149.2978) ccw
  line L162 (-572.135, 168.3619) -> (-546.735, 153.6972)
  arc A230 (-572.135, 168.3619) -> (-579.755, 163.9625) centre (-574.675, 163.9625) ccw
  line L163 (-579.755, 134.6331) -> (-579.755, 163.9625)
  arc A231 (-579.755, 134.6331) -> (-572.135, 130.2337) centre (-574.675, 134.6331) ccw
  line L164 (-586.105, 163.9625) -> (-586.105, 134.6331)
  arc A232 (-586.105, 163.9625) -> (-593.725, 168.3619) centre (-591.185, 163.9625) ccw
  line L165 (-619.125, 153.6972) -> (-593.725, 168.3619)
  arc A233 (-619.125, 153.6972) -> (-619.125, 144.8984) centre (-616.585, 149.2978) ccw
  line L166 (-593.725, 130.2337) -> (-619.125, 144.8984)
  arc A234 (-593.725, 130.2337) -> (-586.105, 134.6331) centre (-591.185, 134.6331) ccw
  line L167 (-568.96, 124.7344) -> (-543.56, 139.3991)
  arc A235 (-535.94, 134.9997) -> (-543.56, 139.3991) centre (-541.02, 134.9997) ccw
  line L168 (-535.94, 134.9997) -> (-535.94, 105.6703)
  arc A236 (-543.56, 101.2709) -> (-535.94, 105.6703) centre (-541.02, 105.6703) ccw
  line L169 (-543.56, 101.2709) -> (-568.96, 115.9356)
  arc A237 (-568.96, 124.7344) -> (-568.96, 115.9356) centre (-566.42, 120.335) ccw
  line L170 (-529.59, 105.6703) -> (-529.59, 134.9997)
  arc A238 (-521.97, 139.3991) -> (-529.59, 134.9997) centre (-524.51, 134.9997) ccw
  line L171 (-521.97, 139.3991) -> (-496.57, 124.7344)
  arc A239 (-496.57, 115.9356) -> (-496.57, 124.7344) centre (-499.11, 120.335) ccw
  line L172 (-496.57, 115.9356) -> (-521.97, 101.2709)
  arc A240 (-529.59, 105.6703) -> (-521.97, 101.2709) centre (-524.51, 105.6703) ccw
  line L173 (-493.395, 130.2337) -> (-518.795, 144.8984)
  arc A241 (-518.795, 153.6972) -> (-518.795, 144.8984) centre (-516.255, 149.2978) ccw
  line L174 (-518.795, 153.6972) -> (-493.395, 168.3619)
  arc A242 (-485.775, 163.9625) -> (-493.395, 168.3619) centre (-490.855, 163.9625) ccw
  line L175 (-485.775, 163.9625) -> (-485.775, 134.6331)
  arc A243 (-493.395, 130.2337) -> (-485.775, 134.6331) centre (-490.855, 134.6331) ccw
  line L176 (-496.57, 173.8612) -> (-521.97, 159.1965)
  arc A244 (-529.59, 163.5959) -> (-521.97, 159.1965) centre (-524.51, 163.5959) ccw
  line L177 (-529.59, 163.5959) -> (-529.59, 192.9253)
  arc A245 (-521.97, 197.3247) -> (-529.59, 192.9253) centre (-524.51, 192.9253) ccw
  line L178 (-521.97, 197.3247) -> (-496.57, 182.66)
  arc A246 (-496.57, 173.8612) -> (-496.57, 182.66) centre (-499.11, 178.2606) ccw
  line L179 (-535.94, 192.9253) -> (-535.94, 163.5959)
  arc A247 (-543.56, 159.1965) -> (-535.94, 163.5959) centre (-541.02, 163.5959) ccw
  line L180 (-543.56, 159.1965) -> (-568.96, 173.8612)
  arc A248 (-568.96, 182.66) -> (-568.96, 173.8612) centre (-566.42, 178.2606) ccw
  line L181 (-568.96, 182.66) -> (-543.56, 197.3247)
  arc A249 (-535.94, 192.9253) -> (-543.56, 197.3247) centre (-541.02, 192.9253) ccw
  circle A250 centre (-582.93, 178.2606) radius 11.43 construction
  arc A251 (-579.755, 134.6331) -> (-572.135, 130.2337) centre (-574.675, 134.6331) ccw
  line L182 (-546.735, 144.8984) -> (-572.135, 130.2337)
  arc A252 (-546.735, 144.8984) -> (-546.735, 153.6972) centre (-549.275, 149.2978) ccw
  line L183 (-572.135, 168.3619) -> (-546.735, 153.6972)
  line L184 (-579.755, 134.6331) -> (-579.755, 163.9625)
  arc A253 (-572.135, 168.3619) -> (-579.755, 163.9625) centre (-574.675, 163.9625) ccw
  arc A254 (-543.56, 159.1965) -> (-535.94, 163.5959) centre (-541.02, 163.5959) ccw
  line L185 (-535.94, 192.9253) -> (-535.94, 163.5959)
  arc A255 (-535.94, 192.9253) -> (-543.56, 197.3247) centre (-541.02, 192.9253) ccw
  line L186 (-568.96, 182.66) -> (-543.56, 197.3247)
  line L187 (-543.56, 159.1965) -> (-568.96, 173.8612)
  arc A256 (-568.96, 182.66) -> (-568.96, 173.8612) centre (-566.42, 178.2606) ccw
  arc A257 (-546.735, 202.8239) -> (-546.735, 211.6228) centre (-549.275, 207.2233) ccw
  line L188 (-572.135, 226.2874) -> (-546.735, 211.6228)
  arc A258 (-572.135, 226.2874) -> (-579.755, 221.888) centre (-574.675, 221.888) ccw
  line L189 (-579.755, 192.5586) -> (-579.755, 221.888)
  line L190 (-546.735, 202.8239) -> (-572.135, 188.1592)
  arc A259 (-579.755, 192.5586) -> (-572.135, 188.1592) centre (-574.675, 192.5586) ccw
  arc A260 (-586.105, 221.888) -> (-593.725, 226.2874) centre (-591.185, 221.888) ccw
  line L191 (-619.125, 211.6228) -> (-593.725, 226.2874)
  arc A261 (-619.125, 211.6228) -> (-619.125, 202.8239) centre (-616.585, 207.2233) ccw
  line L192 (-593.725, 188.1592) -> (-619.125, 202.8239)
  line L193 (-586.105, 221.888) -> (-586.105, 192.5586)
  arc A262 (-593.725, 188.1592) -> (-586.105, 192.5586) centre (-591.185, 192.5586) ccw
  arc A263 (-622.3, 197.3247) -> (-629.92, 192.9253) centre (-624.84, 192.9253) ccw
  line L194 (-629.92, 163.5959) -> (-629.92, 192.9253)
  arc A264 (-629.92, 163.5959) -> (-622.3, 159.1965) centre (-624.84, 163.5959) ccw
  line L195 (-596.9, 173.8612) -> (-622.3, 159.1965)
  line L196 (-622.3, 197.3247) -> (-596.9, 182.66)
  arc A265 (-596.9, 173.8612) -> (-596.9, 182.66) centre (-599.44, 178.2606) ccw
  circle A266 centre (-633.095, 207.2233) radius 11.43 construction
  line L197 (-596.9, 231.7867) -> (-622.3, 217.122)
  arc A267 (-596.9, 231.7867) -> (-596.9, 240.5855) centre (-599.44, 236.1861) ccw
  line L198 (-622.3, 255.2502) -> (-596.9, 240.5855)
  arc A268 (-622.3, 255.2502) -> (-629.92, 250.8508) centre (-624.84, 250.8508) ccw
  line L199 (-629.92, 221.5214) -> (-629.92, 250.8508)
  arc A269 (-629.92, 221.5214) -> (-622.3, 217.122) centre (-624.84, 221.5214) ccw
  line L200 (-636.27, 250.8508) -> (-636.27, 221.5214)
  arc A270 (-636.27, 250.8508) -> (-643.89, 255.2502) centre (-641.35, 250.8508) ccw
  line L201 (-669.29, 240.5855) -> (-643.89, 255.2502)
  arc A271 (-669.29, 240.5855) -> (-669.29, 231.7867) centre (-666.75, 236.1861) ccw
  line L202 (-643.89, 217.122) -> (-669.29, 231.7867)
  arc A272 (-643.89, 217.122) -> (-636.27, 221.5214) centre (-641.35, 221.5214) ccw
  circle A273 centre (-683.26, 236.1861) radius 11.43 construction
  line L203 (-647.065, 260.7495) -> (-672.465, 246.0848)
  arc A274 (-647.065, 260.7495) -> (-647.065, 269.5483) centre (-649.605, 265.1489) ccw
  line L204 (-672.465, 284.213) -> (-647.065, 269.5483)
  arc A275 (-672.465, 284.213) -> (-680.085, 279.8136) centre (-675.005, 279.8136) ccw
  line L205 (-680.085, 250.4842) -> (-680.085, 279.8136)
  arc A276 (-680.085, 250.4842) -> (-672.465, 246.0848) centre (-675.005, 250.4842) ccw
  line L206 (-686.435, 279.8136) -> (-686.435, 250.4842)
  arc A277 (-686.435, 279.8136) -> (-694.055, 284.213) centre (-691.515, 279.8136) ccw
  line L207 (-719.455, 269.5483) -> (-694.055, 284.213)
  arc A278 (-719.455, 269.5483) -> (-719.455, 260.7495) centre (-716.915, 265.1489) ccw
  line L208 (-694.055, 246.0848) -> (-719.455, 260.7495)
  arc A279 (-694.055, 246.0848) -> (-686.435, 250.4842) centre (-691.515, 250.4842) ccw
  line L209 (-672.465, 226.2874) -> (-647.065, 211.6228)
  arc A280 (-672.465, 226.2874) -> (-680.085, 221.888) centre (-675.005, 221.888) ccw
  line L210 (-680.085, 192.5586) -> (-680.085, 221.888)
  arc A281 (-680.085, 192.5586) -> (-672.465, 188.1592) centre (-675.005, 192.5586) ccw
  line L211 (-647.065, 202.8239) -> (-672.465, 188.1592)
  arc A282 (-647.065, 202.8239) -> (-647.065, 211.6228) centre (-649.605, 207.2233) ccw
  circle A283 centre (-683.26, 294.1117) radius 11.43 construction
  line L212 (-672.465, 284.213) -> (-647.065, 269.5483)
  arc A284 (-647.065, 260.7495) -> (-647.065, 269.5483) centre (-649.605, 265.1489) ccw
  line L213 (-647.065, 260.7495) -> (-672.465, 246.0848)
  arc A285 (-680.085, 250.4842) -> (-672.465, 246.0848) centre (-675.005, 250.4842) ccw
  line L214 (-680.085, 250.4842) -> (-680.085, 279.8136)
  arc A286 (-672.465, 284.213) -> (-680.085, 279.8136) centre (-675.005, 279.8136) ccw
  line L215 (-669.29, 298.5111) -> (-643.89, 313.1758)
  arc A287 (-636.27, 308.7764) -> (-643.89, 313.1758) centre (-641.35, 308.7764) ccw
  line L216 (-636.27, 308.7764) -> (-636.27, 279.447)
  arc A288 (-643.89, 275.0476) -> (-636.27, 279.447) centre (-641.35, 279.447) ccw
  line L217 (-643.89, 275.0476) -> (-669.29, 289.7123)
  arc A289 (-669.29, 298.5111) -> (-669.29, 289.7123) centre (-666.75, 294.1117) ccw
  line L218 (-680.085, 308.4098) -> (-680.085, 337.7391)
  arc A290 (-672.465, 342.1386) -> (-680.085, 337.7391) centre (-675.005, 337.7391) ccw
  line L219 (-672.465, 342.1386) -> (-647.065, 327.4739)
  arc A291 (-647.065, 318.675) -> (-647.065, 327.4739) centre (-649.605, 323.0744) ccw
  line L220 (-647.065, 318.675) -> (-672.465, 304.0103)
  arc A292 (-680.085, 308.4098) -> (-672.465, 304.0103) centre (-675.005, 308.4098) ccw
  line L221 (-694.055, 304.0103) -> (-719.455, 318.675)
  arc A293 (-719.455, 327.4739) -> (-719.455, 318.675) centre (-716.915, 323.0744) ccw
  line L222 (-719.455, 327.4739) -> (-694.055, 342.1386)
  arc A294 (-686.435, 337.7391) -> (-694.055, 342.1386) centre (-691.515, 337.7391) ccw
  line L223 (-686.435, 337.7391) -> (-686.435, 308.4098)
  arc A295 (-694.055, 304.0103) -> (-686.435, 308.4098) centre (-691.515, 308.4098) ccw
  line L224 (-697.23, 289.7123) -> (-722.63, 275.0476)
  arc A296 (-730.25, 279.447) -> (-722.63, 275.0476) centre (-725.17, 279.447) ccw
  line L225 (-730.25, 279.447) -> (-730.25, 308.7764)
  arc A297 (-722.63, 313.1758) -> (-730.25, 308.7764) centre (-725.17, 308.7764) ccw
  line L226 (-722.63, 313.1758) -> (-697.23, 298.5111)
  arc A298 (-697.23, 289.7123) -> (-697.23, 298.5111) centre (-699.77, 294.1117) ccw
  circle A299 centre (-683.26, 352.0372) radius 11.43 construction
  line L227 (-672.465, 342.1386) -> (-647.065, 327.4739)
  arc A300 (-647.065, 318.675) -> (-647.065, 327.4739) centre (-649.605, 323.0744) ccw
  line L228 (-647.065, 318.675) -> (-672.465, 304.0103)
  arc A301 (-680.085, 308.4098) -> (-672.465, 304.0103) centre (-675.005, 308.4098) ccw
  line L229 (-680.085, 308.4098) -> (-680.085, 337.7391)
  circle A302 centre (-683.26, 352.0372) radius 11.43 construction
  arc A303 (-672.465, 342.1386) -> (-680.085, 337.7391) centre (-675.005, 337.7391) ccw
  line L230 (-669.29, 356.4366) -> (-643.89, 371.1013)
  arc A304 (-636.27, 366.7019) -> (-643.89, 371.1013) centre (-641.35, 366.7019) ccw
  line L231 (-636.27, 366.7019) -> (-636.27, 337.3725)
  arc A305 (-643.89, 332.9731) -> (-636.27, 337.3725) centre (-641.35, 337.3725) ccw
  line L232 (-643.89, 332.9731) -> (-669.29, 347.6378)
  circle A306 centre (-683.26, 352.0372) radius 11.43 construction
  arc A307 (-669.29, 356.4366) -> (-669.29, 347.6378) centre (-666.75, 352.0372) ccw
  line L233 (-680.085, 366.3353) -> (-680.085, 395.6647)
  arc A308 (-672.465, 400.0641) -> (-680.085, 395.6647) centre (-675.005, 395.6647) ccw
  line L234 (-672.465, 400.0641) -> (-647.065, 385.3994)
  arc A309 (-647.065, 376.6006) -> (-647.065, 385.3994) centre (-649.605, 381) ccw
  line L235 (-647.065, 376.6006) -> (-672.465, 361.9359)
  circle A310 centre (-683.26, 352.0372) radius 11.43 construction
  arc A311 (-680.085, 366.3353) -> (-672.465, 361.9359) centre (-675.005, 366.3353) ccw
  line L236 (-694.055, 361.9359) -> (-719.455, 376.6006)
  arc A312 (-719.455, 385.3994) -> (-719.455, 376.6006) centre (-716.915, 381) ccw
  line L237 (-719.455, 385.3994) -> (-694.055, 400.0641)
  arc A313 (-686.435, 395.6647) -> (-694.055, 400.0641) centre (-691.515, 395.6647) ccw
  line L238 (-686.435, 395.6647) -> (-686.435, 366.3353)
  circle A314 centre (-683.26, 352.0372) radius 11.43 construction
  arc A315 (-694.055, 361.9359) -> (-686.435, 366.3353) centre (-691.515, 366.3353) ccw
  line L239 (-697.23, 347.6378) -> (-722.63, 332.9731)
  arc A316 (-730.25, 337.3725) -> (-722.63, 332.9731) centre (-725.17, 337.3725) ccw
  line L240 (-730.25, 337.3725) -> (-730.25, 366.7019)
  arc A317 (-722.63, 371.1013) -> (-730.25, 366.7019) centre (-725.17, 366.7019) ccw
  line L241 (-722.63, 371.1013) -> (-697.23, 356.4366)
  circle A318 centre (-683.26, 352.0372) radius 11.43 construction
  arc A319 (-697.23, 347.6378) -> (-697.23, 356.4366) centre (-699.77, 352.0372) ccw
  circle A320 centre (-683.26, 409.9628) radius 11.43 construction
  line L242 (-697.23, 405.5634) -> (-722.63, 390.8987)
  line L243 (-722.63, 429.0269) -> (-697.23, 414.3622)
  arc A321 (-722.63, 429.0269) -> (-730.25, 424.6275) centre (-725.17, 424.6275) ccw
  line L244 (-730.25, 395.2981) -> (-730.25, 424.6275)
  arc A322 (-730.25, 395.2981) -> (-722.63, 390.8987) centre (-725.17, 395.2981) ccw
  arc A323 (-697.23, 405.5634) -> (-697.23, 414.3622) centre (-699.77, 409.9628) ccw
  line L245 (-694.055, 419.8614) -> (-719.455, 434.5261)
  line L246 (-686.435, 453.5902) -> (-686.435, 424.2609)
  arc A324 (-686.435, 453.5902) -> (-694.055, 457.9897) centre (-691.515, 453.5902) ccw
  line L247 (-719.455, 443.325) -> (-694.055, 457.9897)
  arc A325 (-719.455, 443.325) -> (-719.455, 434.5261) centre (-716.915, 438.9256) ccw
  arc A326 (-694.055, 419.8614) -> (-686.435, 424.2609) centre (-691.515, 424.2609) ccw
  line L248 (-680.085, 424.2609) -> (-680.085, 453.5902)
  line L249 (-647.065, 434.5261) -> (-672.465, 419.8614)
  arc A327 (-647.065, 434.5261) -> (-647.065, 443.325) centre (-649.605, 438.9256) ccw
  line L250 (-672.465, 457.9897) -> (-647.065, 443.325)
  arc A328 (-672.465, 457.9897) -> (-680.085, 453.5902) centre (-675.005, 453.5902) ccw
  arc A329 (-680.085, 424.2609) -> (-672.465, 419.8614) centre (-675.005, 424.2609) ccw
  line L251 (-669.29, 414.3622) -> (-643.89, 429.0269)
  line L252 (-643.89, 390.8987) -> (-669.29, 405.5634)
  arc A330 (-643.89, 390.8987) -> (-636.27, 395.2981) centre (-641.35, 395.2981) ccw
  line L253 (-636.27, 424.6275) -> (-636.27, 395.2981)
  arc A331 (-636.27, 424.6275) -> (-643.89, 429.0269) centre (-641.35, 424.6275) ccw
  arc A332 (-669.29, 414.3622) -> (-669.29, 405.5634) centre (-666.75, 409.9628) ccw
  line L254 (-672.465, 400.0641) -> (-647.065, 385.3994)
  line L255 (-680.085, 366.3353) -> (-680.085, 395.6647)
  arc A333 (-680.085, 366.3353) -> (-672.465, 361.9359) centre (-675.005, 366.3353) ccw
  line L256 (-647.065, 376.6006) -> (-672.465, 361.9359)
  arc A334 (-647.065, 376.6006) -> (-647.065, 385.3994) centre (-649.605, 381) ccw
  arc A335 (-672.465, 400.0641) -> (-680.085, 395.6647) centre (-675.005, 395.6647) ccw
  circle A336 centre (-683.26, 467.8883) radius 11.43 construction
  line L257 (-636.27, 482.553) -> (-636.27, 453.2236)
  line L258 (-643.89, 448.8242) -> (-669.29, 463.4889)
  arc A337 (-643.89, 448.8242) -> (-636.27, 453.2236) centre (-641.35, 453.2236) ccw
  arc A338 (-669.29, 472.2877) -> (-669.29, 463.4889) centre (-666.75, 467.8883) ccw
  line L259 (-669.29, 472.2877) -> (-643.89, 486.9524)
  arc A339 (-636.27, 482.553) -> (-643.89, 486.9524) centre (-641.35, 482.553) ccw
  line L260 (-672.465, 515.9152) -> (-647.065, 501.2505)
  line L261 (-647.065, 492.4517) -> (-672.465, 477.787)
  arc A340 (-647.065, 492.4517) -> (-647.065, 501.2505) centre (-649.605, 496.8511) ccw
  arc A341 (-680.085, 482.1864) -> (-672.465, 477.787) centre (-675.005, 482.1864) ccw
  line L262 (-680.085, 482.1864) -> (-680.085, 511.5158)
  arc A342 (-672.465, 515.9152) -> (-680.085, 511.5158) centre (-675.005, 511.5158) ccw
  line L263 (-719.455, 501.2505) -> (-694.055, 515.9152)
  line L264 (-686.435, 511.5158) -> (-686.435, 482.1864)
  arc A343 (-686.435, 511.5158) -> (-694.055, 515.9152) centre (-691.515, 511.5158) ccw
  arc A344 (-694.055, 477.787) -> (-686.435, 482.1864) centre (-691.515, 482.1864) ccw
  line L265 (-694.055, 477.787) -> (-719.455, 492.4517)
  arc A345 (-719.455, 501.2505) -> (-719.455, 492.4517) centre (-716.915, 496.8511) ccw
  line L266 (-730.25, 453.2236) -> (-730.25, 482.553)
  line L267 (-722.63, 486.9524) -> (-697.23, 472.2877)
  arc A346 (-722.63, 486.9524) -> (-730.25, 482.553) centre (-725.17, 482.553) ccw
  arc A347 (-697.23, 463.4889) -> (-697.23, 472.2877) centre (-699.77, 467.8883) ccw
  line L268 (-697.23, 463.4889) -> (-722.63, 448.8242)
  arc A348 (-730.25, 453.2236) -> (-722.63, 448.8242) centre (-725.17, 453.2236) ccw
  line L269 (-694.055, 419.8614) -> (-719.455, 434.5261)
  line L270 (-719.455, 443.325) -> (-694.055, 457.9897)
  arc A349 (-719.455, 443.325) -> (-719.455, 434.5261) centre (-716.915, 438.9256) ccw